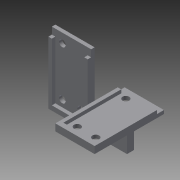
# Autodesk Inventor part: soporte0.2
Saved by Autodesk Inventor 2015 SP1 (Build 190203100, 203)
## iProperties
Created: 2015-06-10
Part Number: soporte0.2
Material: Generic
Document SubType Name: Modeling
Designer: pc
Density: 1 g/cm^3
Appearance: Default
Author: pc
Autodesk Inventor part; units mm, degrees
ref_plane "YZ Plane" through (0, 0, 0) normal (1, 0, 0) x (0, 1, 0)
ref_plane "XZ Plane" through (0, 0, 0) normal (0, 1, 0) x (-1, 0, 0)
ref_plane "XY Plane" through (0, 0, 0) normal (0, 0, 1) x (1, 0, 0)
sketch "Sketch1" plane through (0, 0, 0) normal (0, 0, 1) x (1, 0, 0)
  line L0 (-34, 17) -> (-17, 17)
  line L1 (-17, 17) -> (-17, 30)
  line L2 (-17, 30) -> (0, 30)
  line L3 (0, 30) -> (0, 0)
  line L4 (0, 0) -> (-17, 0)
  line L5 (-17, 0) -> (-17, 14)
  line L6 (-17, 14) -> (-34, 14)
  line L7 (-34, 14) -> (-34, 17)
  dimension "d0" = 17
  dimension "d1" = 13
  dimension "d2" = 17
  dimension "d4" = 17
  dimension "d5" = 14
  dimension "d72" = 3
  constraints: 16 end point, 5 perpendicular, 2 point on line, 1 coincident, 1 horizontal
  measures "d0" distance of L0.start L0.end
  measures "d1" distance of L0.end L1.end
  measures "d2" distance of L1.end L2.end
  measures "d4" distance of L3.end L4.end
  measures "d5" distance of L4.end L5.end
  measures "d72" distance of L6.end L0.start
extrude "Extrusion1" add sketch "Sketch1" along normal blind 30
sketch "Sketch4" plane through (0, 0, 0) normal (0, 0, -1) x (-1, 0, 0)
  line L0 (34, 17) -> (17, 17) projected
  line L1 (17, 17) -> (17, 30) projected
  line L2 (17, 30) -> (0, 30) projected
  line L3 (0, 30) -> (0, 0) projected
  line L4 (0, 0) -> (17, 0) projected
  line L5 (17, 0) -> (17, 14) projected
  line L6 (17, 14) -> (34, 14) projected
  line L7 (34, 14) -> (34, 17) projected
  line L8 (17, 0) -> (0, 0)
  line L9 (0, 0) -> (0, 30)
  line L10 (0, 30) -> (17, 30)
  line L11 (17, 30) -> (17, 0)
  constraints: 8 end point, 2 parallel, 1 horizontal, 1 perpendicular
extrude "Extrusion4" cut sketch "Sketch4" against normal blind 7 contours L11 L5 L4 L3 L2 L1
sketch "Sketch8" plane through (0, 0, 30) normal (0, 0, 1) x (1, 0, 0)
  line L0 (-17, 17) -> (-34, 17) projected
  line L1 (-34, 17) -> (-34, 14) projected
  line L2 (-34, 14) -> (-17, 14) projected
  line L3 (-17, 14) -> (-17, 0) projected
  line L4 (-17, 0) -> (0, 0) projected
  line L5 (0, 0) -> (0, 30) projected
  line L6 (0, 30) -> (-17, 30) projected
  line L7 (-17, 30) -> (-17, 17) projected
  line L8 (-17, 30) -> (0, 30)
  line L9 (0, 30) -> (0, 0)
  line L10 (0, 0) -> (-17, 0)
  line L11 (-17, 0) -> (-17, 30)
  constraints: 8 end point, 2 parallel, 1 horizontal, 1 perpendicular
extrude "Extrusion8" cut sketch "Sketch8" against normal blind 20 contours L7 L6 L5 L4 L3 L11
sketch "Sketch9" plane through (-34, 14, 0) normal (0, -1, 0) x (1, 0, 0)
  line L0 (17, 0) -> (0, 0) projected
  line L1 (17, 0) -> (17, 7) projected
  line L2 (17, 7) -> (17, 10) projected
  line L3 (17, 10) -> (17, 30) projected
  line L4 (0, 30) -> (17, 30) projected
  line L5 (0, 0) -> (0, 30) projected
  line L6 (0, 0) -> (17, 0) projected
  line L7 (0, 30) -> (17, 30) projected
  line L8 (17, 0) -> (0, 0) projected
  line L9 (17, 10) -> (17, 30) projected
  line L10 (17, 30) -> (0, 30) projected
  line L11 (0, 0) -> (0, 30) projected
  line L12 (0, 27) -> (1.5, 27)
  line L13 (1.5, 27) -> (1.5, 2)
  line L14 (1.5, 2) -> (15.5, 2)
  line L15 (17, 27) -> (15.5, 27)
  line L16 (15.5, 27) -> (15.5, 2)
  line L17 (0, 27) -> (0, 30)
  line L18 (17, 30) -> (17, 27)
  point P0 (34, 0)
  dimension "d80" = 1.5
  dimension "d81" = 2
  dimension "d82" = 25
  dimension "d83" = 14
  constraints: 14 end point, 2 collinear, 2 perpendicular, 1 point on line, 1 vertical
  measures "d80" distance of L12.start L12.end
  measures "d81" distance between parallel lines of L0 L14
  measures "d82" distance of L12.end L13.end
  measures "d83" distance of L13.end L14.end
extrude "Extrusion14" cut sketch "Sketch9" against normal blind 1.5 contours L5 L4 L3 L15 L16 L14 L13 L12
sketch "Sketch14" plane through (0, 0, 10) normal (0, 0, 1) x (1, 0, 0)
  line L0 (0, 30) -> (0, 0) projected
  line L1 (-17, 30) -> (0, 30) projected
  line L2 (-17, 17) -> (-17, 30) projected
  line L3 (-17, 14) -> (-17, 17) projected
  line L4 (-17, 0) -> (-17, 14) projected
  line L5 (0, 0) -> (-17, 0) projected
  line L6 (-17, 30) -> (-17, 27)
  line L7 (-17, 30) -> (-17, 17) projected
  line L8 (-15.5, 27) -> (-15.5, 2)
  line L9 (-15.5, 2) -> (-1.5, 2)
  line L10 (-15.5, 27) -> (-17, 27)
  line L11 (-17, 30) -> (0, 30)
  line L12 (0, 30) -> (-17, 30) projected
  line L13 (-17, 0) -> (0, 0) projected
  line L14 (0, 27) -> (0, 30)
  line L15 (-1.5, 27) -> (-1.5, 2)
  line L16 (-1.5, 27) -> (0, 27)
  line L17 (0, 30) -> (0, 0) projected
  point P0 (0, 30)
  point P1 (-16.25, 27)
  point P2 (-0.75, 27)
  dimension "d87" = 1.5
  dimension "d88" = 2
  dimension "d89" = 25
  dimension "d91" = 1.5
  dimension "d93" = 14
  constraints: 16 end point, 3 point on line, 2 midpoint, 1 horizontal, 1 horizontal alignment, 1 perpendicular, 1 vertical
  measures "d87" distance of L8.start L6.end
  measures "d88" distance between parallel lines of L5 L9
  measures "d89" distance of L8.start L8.end
  measures "d91" distance of L16.start L16.end
  measures "d93" distance of L8.end L9.end
extrude "Extrusion15" cut sketch "Sketch14" against normal blind 1.5 contours L0 L16 L15 L9 L8 L10 L2 L1
sketch "Sketch15" plane through (-34, 15.5, 0) normal (0, -1, 0) x (1, 0, 0)
  line L0 (0, 30) -> (17, 30) projected
  line L1 (0, 27) -> (0, 30) projected
  line L2 (1.5, 27) -> (0, 27) projected
  line L3 (1.5, 2) -> (1.5, 27) projected
  line L4 (15.5, 2) -> (1.5, 2) projected
  line L5 (15.5, 27) -> (15.5, 2) projected
  line L6 (17, 27) -> (15.5, 27) projected
  line L7 (17, 30) -> (17, 27) projected
  circle A0 centre (4.5, 26) radius 1.45
  circle A1 centre (4.5, 5) radius 1.45
  circle A2 centre (12.5, 5) radius 1.45
  point P0 (34, 0)
  dimension "d96" = 2.9
  dimension "d97" = 21
  dimension "d98" = 8
  dimension "d99" = 3
  dimension "d100" = 3
  constraints: 3 centre point, 2 equal radius, 1 horizontal alignment, 1 vertical alignment
  measures "d96" diameter of A0
  measures "d97" distance of A1.centre A0.centre
  measures "d98" distance of A2.centre A1.centre
  measures "d99" distance from line of L4 A1.centre
  measures "d100" distance from line of L3 A1.centre
extrude "Extrusion16" cut sketch "Sketch15" against normal through all contours A0 | A1 | A2
sketch "Sketch16" plane through (0, 0, 8.5) normal (0, 0, 1) x (1, 0, 0)
  line L0 (-17, 27) -> (-17, 30) projected
  line L1 (-15.5, 27) -> (-17, 27) projected
  line L2 (-15.5, 2) -> (-15.5, 27) projected
  line L3 (-1.5, 2) -> (-15.5, 2) projected
  line L4 (-1.5, 27) -> (-1.5, 2) projected
  line L5 (0, 27) -> (-1.5, 27) projected
  line L6 (0, 30) -> (0, 27) projected
  line L7 (-17, 30) -> (0, 30) projected
  circle A0 centre (-12.5, 5) radius 1.45
  circle A1 centre (-4.5, 5) radius 1.45
  circle A2 centre (-12.5, 26) radius 1.45
  point P0 (0, 0)
  dimension "d103" = 3
  dimension "d104" = 3
  dimension "d105" = 8
  dimension "d106" = 21
  dimension "d107" = 2.9
  constraints: 3 centre point, 2 equal radius, 1 horizontal alignment, 1 vertical alignment
  measures "d103" distance from line of L3 A0.centre
  measures "d104" distance from line of L2 A0.centre
  measures "d105" distance of A1.centre A0.centre
  measures "d106" distance of A2.centre A0.centre
  measures "d107" diameter of A2
extrude "Extrusion18" cut sketch "Sketch16" against normal through all contours A0 | A1 | A2
sketch "Sketch17" plane through (-17, 14, 0) normal (1, 0, 0) x (0, 0, -1)
  line L0 (0, 0) -> (-7, 0) projected
  line L1 (0, 3) -> (0, 0) projected
  line L2 (0, 3) -> (-7, 3) projected
  line L3 (-7, 3) -> (-7, 0) projected
  line L4 (0, 0) -> (-7, 0)
  line L5 (-7, 0) -> (-7, 3)
  line L6 (-7, 3) -> (0, 3)
  line L7 (0, 3) -> (0, 0)
  point P0 (0, -14)
  dimension "d54" = 2.7
  dimension "d55" = 21
  dimension "d56" = 3
  dimension "d57" = 8
  dimension "d58" = 3
  dimension "d59" = 2.8
  dimension "d60" = 21
  dimension "d61" = 8
  dimension "d62" = 3
  dimension "d63" = 3
  constraints: 8 end point, 2 parallel, 1 horizontal, 1 perpendicular
extrude "Extrusion19" add sketch "Sketch17" along normal up to surface (17 mm away) from surface at 0
sketch "Sketch13" plane through (-17, 14, 0) normal (1, 0, 0) x (0, 0, -1)
  line L0 (0, 0) -> (-7, 0) projected
  line L1 (0, 3) -> (0, 0) projected
  line L2 (0, 3) -> (-7, 3) projected
  line L3 (-7, 3) -> (-7, 0) projected
  line L4 (0, 0) -> (-7, 0)
  line L5 (-7, 0) -> (-7, 3)
  line L6 (-7, 3) -> (0, 3)
  line L7 (0, 3) -> (0, 0)
  point P0 (0, -14)
  constraints: 8 end point, 2 parallel, 1 horizontal, 1 perpendicular
body "Solid1"
